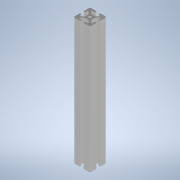
# Autodesk Inventor part: 40-4040-25-CL
Saved by Autodesk Inventor 2021 (Build 250183000, 183)
## iProperties
Category: PARTsolutions
Company: 8020
Part Number: 40-4040-25-CL
Material: Aluminum 6061
Catalog Web Link: www.cadenas.de
Description: 40-4040, 40-4040-Black-T-Slotted Profile - 40 Series
Vendor: 8020
Document SubType Name: Modeling
Designer: partserver
Manufacturer: 8020
Mass: 59.5796 g
Surface Area: 99.7707 cm^2
Volume: 22.0665 cm^3
Density: 2.7 g/cm^3
Appearance: Aluminum - Flat
PSOL_IDENT_0: {$CADENAS_DATA\23d-libs\8020\metric\profiles\40_series\40_4040.prj},191 {VTYP=3D},{NB=40-4040-25-CL}
PSOL_IDENT_1: ,{LINA=40-4040-25},{NN=40-4040, 40-4040-Black},{DATE=31.07.2020 09:21:33},{GEOMDATE=27.02.2018 07:10
PSOL_IDENT_2: :12},{VERSION=},{LINEID=10},{WBVAR=FINISH,LS,L},{WBNUMERIC=L}  {NB=40-4040-25-CL},{LINA=40-4040-25},
PSOL_IDENT_3: {KT=DUMMY},{PN=40-4040-25},{PN1=40-4040},{SERIES=40-4040},{MAT=6105-T5 Aluminum},{FINISH=CA},{LS=-CL
PSOL_IDENT_4: },{L=25.00},{W=2.3624},{LALG=[25:6000/0.05]},{MIX=13.7871},{MIY=13.7871},{EA=8.7804},{CLR=.75,.75,.7
PSOL_IDENT_5: 5}
NB: 40-4040-25-CL
NN: 40-4040, 40-4040-Black
NT: T-Slotted Profile - 40 Series
NBSYN: $PN.$LS.
LINA: 40-4040-25
CATALOG: 80/20
PN: 40-4040-25
SERIES: 40-4040
MAT: 6105-T5 Aluminum
FINISH: Clear Anodize
LS: Custom Length
L: 25
W: 2.3624
MIX: 13.7871
MIY: 13.7871
EA: 8.7804
SUPPLIER: 8020
ARTICLENO: 40-4040-25-CL
BOMINFO: 40-4040-25
CREATOR: CADENAS GmbH
Title: 40-4040-25
Author: Cadenas PARTsolutions
Comments: T-Slotted Profile - 40 Series
Autodesk Inventor part; units mm, degrees
ref_plane "YZ Plane" through (0, 0, 0) normal (1, 0, 0) x (0, 1, 0)
ref_plane "XZ Plane" through (0, 0, 0) normal (0, 1, 0) x (-1, 0, 0)
ref_plane "XY Plane" through (0, 0, 0) normal (0, 0, 1) x (1, 0, 0)
sketch "Sketch_1" plane through (0, 0, 0) normal (0, 0, 1) x (1, 0, 0)
  line L0 (-20, 16.83) -> (-20, 5.6904)
  arc A0 (-20, 5.6904) -> (-18.43, 4.1204) centre (-18.43, 5.6904) ccw
  line L1 (-18.43, 4.1204) -> (-17.25, 4.1204)
  arc A1 (-17.25, 4.1204) -> (-15.68, 5.6904) centre (-17.25, 5.6904) ccw
  line L2 (-15.68, 5.6904) -> (-15.68, 8.7154)
  arc A2 (-14.11, 10.2854) -> (-15.68, 8.7154) centre (-14.11, 8.7154) ccw
  line L3 (-14.11, 10.2854) -> (-13.6549, 10.2854)
  arc A3 (-13.1175, 10.0628) -> (-13.6549, 10.2854) centre (-13.6549, 9.5254) ccw
  line L4 (-13.1175, 10.0628) -> (-9.1098, 6.0551)
  arc A4 (-7.685, 2.6153) -> (-9.1098, 6.0551) centre (-12.5496, 2.6153) ccw
  line L5 (-7.685, 2.6153) -> (-7.685, -2.6153)
  arc A5 (-9.1098, -6.0551) -> (-7.685, -2.6153) centre (-12.5496, -2.6153) ccw
  line L6 (-9.1098, -6.0551) -> (-13.1175, -10.0628)
  arc A6 (-13.6549, -10.2854) -> (-13.1175, -10.0628) centre (-13.6549, -9.5254) ccw
  line L7 (-13.6549, -10.2854) -> (-14.11, -10.2854)
  arc A7 (-15.68, -8.7154) -> (-14.11, -10.2854) centre (-14.11, -8.7154) ccw
  line L8 (-15.68, -8.7154) -> (-15.68, -5.6904)
  arc A8 (-15.68, -5.6904) -> (-17.25, -4.1204) centre (-17.25, -5.6904) ccw
  line L9 (-17.25, -4.1204) -> (-18.43, -4.1204)
  arc A9 (-18.43, -4.1204) -> (-20, -5.6904) centre (-18.43, -5.6904) ccw
  line L10 (-20, -5.6904) -> (-20, -16.83)
  arc A10 (-20, -16.83) -> (-16.83, -20) centre (-16.83, -16.83) ccw
  line L11 (-16.83, -20) -> (-5.6904, -20)
  arc A11 (-5.6904, -20) -> (-4.1204, -18.43) centre (-5.6904, -18.43) ccw
  line L12 (-4.1204, -18.43) -> (-4.1204, -17.25)
  arc A12 (-4.1204, -17.25) -> (-5.6904, -15.68) centre (-5.6904, -17.25) ccw
  line L13 (-5.6904, -15.68) -> (-8.7154, -15.68)
  arc A13 (-10.2854, -14.11) -> (-8.7154, -15.68) centre (-8.7154, -14.11) ccw
  line L14 (-10.2854, -14.11) -> (-10.2854, -13.6549)
  arc A14 (-10.0628, -13.1175) -> (-10.2854, -13.6549) centre (-9.5254, -13.6549) ccw
  line L15 (-10.0628, -13.1175) -> (-6.0551, -9.1098)
  arc A15 (-2.6153, -7.685) -> (-6.0551, -9.1098) centre (-2.6153, -12.5496) ccw
  line L16 (-2.6153, -7.685) -> (2.6153, -7.685)
  arc A16 (6.0551, -9.1098) -> (2.6153, -7.685) centre (2.6153, -12.5496) ccw
  line L17 (6.0551, -9.1098) -> (10.0628, -13.1175)
  arc A17 (10.2854, -13.6549) -> (10.0628, -13.1175) centre (9.5254, -13.6549) ccw
  line L18 (10.2854, -13.6549) -> (10.2854, -14.11)
  arc A18 (8.7154, -15.68) -> (10.2854, -14.11) centre (8.7154, -14.11) ccw
  line L19 (8.7154, -15.68) -> (5.6904, -15.68)
  arc A19 (5.6904, -15.68) -> (4.1204, -17.25) centre (5.6904, -17.25) ccw
  line L20 (4.1204, -17.25) -> (4.1204, -18.43)
  arc A20 (4.1204, -18.43) -> (5.6904, -20) centre (5.6904, -18.43) ccw
  line L21 (5.6904, -20) -> (16.83, -20)
  arc A21 (16.83, -20) -> (20, -16.83) centre (16.83, -16.83) ccw
  line L22 (20, -16.83) -> (20, -5.6904)
  arc A22 (20, -5.6904) -> (18.43, -4.1204) centre (18.43, -5.6904) ccw
  line L23 (18.43, -4.1204) -> (17.25, -4.1204)
  arc A23 (17.25, -4.1204) -> (15.68, -5.6904) centre (17.25, -5.6904) ccw
  line L24 (15.68, -5.6904) -> (15.68, -8.7154)
  arc A24 (14.11, -10.2854) -> (15.68, -8.7154) centre (14.11, -8.7154) ccw
  line L25 (14.11, -10.2854) -> (13.6549, -10.2854)
  arc A25 (13.1175, -10.0628) -> (13.6549, -10.2854) centre (13.6549, -9.5254) ccw
  line L26 (13.1175, -10.0628) -> (9.1098, -6.0551)
  arc A26 (7.685, -2.6153) -> (9.1098, -6.0551) centre (12.5496, -2.6153) ccw
  line L27 (7.685, -2.6153) -> (7.685, 2.6153)
  arc A27 (9.1098, 6.0551) -> (7.685, 2.6153) centre (12.5496, 2.6153) ccw
  line L28 (9.1098, 6.0551) -> (13.1175, 10.0628)
  arc A28 (13.6549, 10.2854) -> (13.1175, 10.0628) centre (13.6549, 9.5254) ccw
  line L29 (13.6549, 10.2854) -> (14.11, 10.2854)
  arc A29 (15.68, 8.7154) -> (14.11, 10.2854) centre (14.11, 8.7154) ccw
  line L30 (15.68, 8.7154) -> (15.68, 5.6904)
  arc A30 (15.68, 5.6904) -> (17.25, 4.1204) centre (17.25, 5.6904) ccw
  line L31 (17.25, 4.1204) -> (18.43, 4.1204)
  arc A31 (18.43, 4.1204) -> (20, 5.6904) centre (18.43, 5.6904) ccw
  line L32 (20, 5.6904) -> (20, 16.83)
  arc A32 (20, 16.83) -> (16.83, 20) centre (16.83, 16.83) ccw
  line L33 (16.83, 20) -> (5.6904, 20)
  arc A33 (5.6904, 20) -> (4.1204, 18.43) centre (5.6904, 18.43) ccw
  line L34 (4.1204, 18.43) -> (4.1204, 17.25)
  arc A34 (4.1204, 17.25) -> (5.6904, 15.68) centre (5.6904, 17.25) ccw
  line L35 (5.6904, 15.68) -> (8.7154, 15.68)
  arc A35 (10.2854, 14.11) -> (8.7154, 15.68) centre (8.7154, 14.11) ccw
  line L36 (10.2854, 14.11) -> (10.2854, 13.6549)
  arc A36 (10.0628, 13.1175) -> (10.2854, 13.6549) centre (9.5254, 13.6549) ccw
  line L37 (10.0628, 13.1175) -> (6.0551, 9.1098)
  arc A37 (2.6153, 7.685) -> (6.0551, 9.1098) centre (2.6153, 12.5496) ccw
  line L38 (2.6153, 7.685) -> (-2.6153, 7.685)
  arc A38 (-6.0551, 9.1098) -> (-2.6153, 7.685) centre (-2.6153, 12.5496) ccw
  line L39 (-6.0551, 9.1098) -> (-10.0628, 13.1175)
  arc A39 (-10.2854, 13.6549) -> (-10.0628, 13.1175) centre (-9.5254, 13.6549) ccw
  line L40 (-10.2854, 13.6549) -> (-10.2854, 14.11)
  arc A40 (-8.7154, 15.68) -> (-10.2854, 14.11) centre (-8.7154, 14.11) ccw
  line L41 (-8.7154, 15.68) -> (-5.6904, 15.68)
  arc A41 (-5.6904, 15.68) -> (-4.1204, 17.25) centre (-5.6904, 17.25) ccw
  line L42 (-4.1204, 17.25) -> (-4.1204, 18.43)
  arc A42 (-4.1204, 18.43) -> (-5.6904, 20) centre (-5.6904, 18.43) ccw
  line L43 (-5.6904, 20) -> (-16.83, 20)
  arc A43 (-16.83, 20) -> (-20, 16.83) centre (-16.83, 16.83) ccw
  circle A44 centre (0, 0) radius 3.4
  constraints: 88 end point, 88 point on circle, 45 centre point
extrude "Extrusion1" add sketch "Sketch_1" against normal blind 25
ref_plane "to_parts_XY" through (0, 0, -12.5) normal (0, 0, 1) x (1, 0, 0)
ref_plane "to_parts_YZ" through (0, 0, -12.5) normal (1, 0, 0) x (0, 1, 0)
ref_plane "to_parts_ZX" through (0, 0, -12.5) normal (0, 1, 0) x (0, 0, 1)
thicken "Thicken1" operation add thickness 0.4 both sides no extend neighbours yes toward (0, 0, -1) faces at (-13.8451, -14.9018, -25)
thicken "Thicken2" operation add thickness 279.4 both sides no extend neighbours yes toward (0, 0, -1) faces at (-14.9018, 13.8451, -25.4)
body "Solid1"
